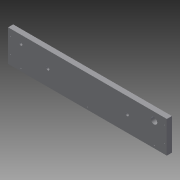
# Autodesk Inventor part: licht_50_top
Saved by Autodesk Inventor 2015 (Build 190159000, 159)
## iProperties
Created: 2018-01-11
Part Number: licht_50_top
Material: Generisch
Document SubType Name: Blech
Designer: schueler
Density: 1 g/cm^3
Sheet Metal Rule: Standard_mm
Appearance: Vorgabe
Author: schueler
Autodesk Inventor part; units mm, degrees
ref_plane "YZ Plane" through (0, 0, 0) normal (1, 0, 0) x (0, 1, 0)
ref_plane "XZ Plane" through (0, 0, 0) normal (0, 1, 0) x (-1, 0, 0)
ref_plane "XY Plane" through (0, 0, 0) normal (0, 0, 1) x (1, 0, 0)
sketch "Skizze1" plane through (0, 0, 0) normal (0, 1, 0) x (-1, 0, 0)
  line L0 (0, 0) -> (500, 0)
  line L1 (500, 0) -> (500, -100)
  line L2 (500, -100) -> (0, -100)
  line L3 (0, -100) -> (0, 0)
  line L4 (125, 0) -> (125, -100) construction
  line L5 (375, 0) -> (375, -100) construction
  line L6 (250, 0) -> (250, -100) construction
  line L7 (0, -50) -> (500, -50) construction
  line L8 (0, -25) -> (500, -25) construction
  line L9 (40, 0) -> (40, -100) construction
  line L10 (460, 0) -> (460, -100) construction
  circle A0 centre (40, -25) radius 10
  circle A1 centre (460, -25) radius 3.5
  circle A2 centre (125, -50) radius 2.5
  circle A3 centre (375, -50) radius 2.5
  line L11 (0, -92) -> (500, -92) construction
  circle A4 centre (40, -92) radius 1.5
  circle A5 centre (250, -92) radius 1.5
  circle A6 centre (460, -92) radius 1.5
  line L12 (8, 0) -> (8, -100) construction
  line L13 (492, 0) -> (492, -100) construction
  line L14 (0, -20) -> (500, -20) construction
  line L15 (0, -70) -> (500, -70) construction
  circle A7 centre (8, -20) radius 1.5
  circle A8 centre (8, -70) radius 1.5
  circle A9 centre (492, -70) radius 1.5
  circle A10 centre (492, -20) radius 1.5
  dimension "d2" = 500
  dimension "d3" = 100
  dimension "d4" = 125
  dimension "d5" = 125
  dimension "d6" = 25
  dimension "d7" = 40
  dimension "d8" = 40
  dimension "d9" = 20
  dimension "d10" = 7
  dimension "d11" = 5
  dimension "d12" = 5
  dimension "d15" = 8
  dimension "d16" = 3
  dimension "d17" = 3
  dimension "d18" = 3
  dimension "d19" = 8
  dimension "d20" = 8
  dimension "d21" = 20
  dimension "d22" = 50
  dimension "d23" = 3
  dimension "d24" = 3
  dimension "d25" = 3
  dimension "d26" = 3
  constraints: 28 end point, 26 point on line, 11 centre point, 7 vertical, 5 midpoint, 4 perpendicular, 2 coincident, 1 parallel, 20 other
  measures "d2" distance of L1.end L3.start
  measures "d3" distance of L1.start L1.end
  measures "d4" distance of L6.start L4.start
  measures "d5" distance of L5.start L6.start
  measures "d6" distance of L8.start L3.end
  measures "d7" distance of L3.end L9.start
  measures "d8" distance of L1.start L10.start
  measures "d9" diameter of A0
  measures "d10" diameter of A1
  measures "d11" diameter of A2
  measures "d12" diameter of A3
  measures "d15" distance of L3.start L11.start
  measures "d16" diameter of A4
  measures "d17" diameter of A5
  measures "d18" diameter of A6
  measures "d19" distance of L3.end L12.start
  measures "d20" distance of L1.start L13.start
  measures "d21" distance of L1.start L14.end
  measures "d22" distance of L15.end L14.end
  measures "d23" diameter of A7
  measures "d24" diameter of A8
  measures "d25" diameter of A9
  measures "d26" diameter of A10
extrude "Extrusion2" add sketch "Skizze1" along normal blind 16
sketch "Skizze2" plane through (0, 0, 0) normal (0, -1, 0) x (1, 0, 0)
  circle A0 centre (-375, -50) radius 2.5 projected
  circle A1 centre (-125, -50) radius 2.5 projected
  circle A2 centre (-460, -25) radius 3.5 projected
  point P0 (0, 0)
hole "Bohrung1" at (-375, 0, -50) at (-125, 0, -50) at (-460, 0, -25) direction (0, 1, 0) diameter 10 depth 12 tip angle 118
sketch "Skizze3" plane through (0, 16, 0) normal (0, 1, 0) x (1, 0, 0)
  circle A0 centre (-8, 20) radius 1.5 projected
  circle A1 centre (-8, 70) radius 1.5 projected
  circle A2 centre (-40, 92) radius 1.5 projected
  circle A3 centre (-250, 92) radius 1.5 projected
  circle A4 centre (-460, 92) radius 1.5 projected
  circle A5 centre (-492, 70) radius 1.5 projected
  circle A6 centre (-492, 20) radius 1.5 projected
  point P0 (0, 0)
hole "Bohrung2" at (-8, 16, -20) at (-8, 16, -70) at (-40, 16, -92) at (-250, 16, -92) at (-460, 16, -92) at (-492, 16, -70) at (-492, 16, -20) direction (0, -1, 0) diameter 3 depth 8 tip angle 118 countersink diameter 8 countersink angle 90
equation "\"Biegeradius\" = Stärke"
equation "\"BreiteBiegungsfreistellung\" = Stärke"
equation "\"TiefeBiegungsfreistellung\" = 0.5 * Stärke"
equation "\"GrößeEckenfreistellung\" = 4 * Stärke"
equation "\"MinimalRest\" = 2 * Stärke"
equation "\"Übergangsradius\" = Biegeradius"
equation "\"JacobiRadiusGröße\" = Biegeradius"
equation "\"Abstandsgröße\" = Stärke"
equation "\"Stärke\" = 0.5"
